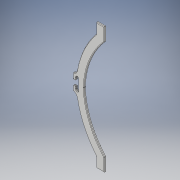
# Autodesk Inventor part: Baseplate_aussen_unten
Saved by Autodesk Inventor 2018 (Build 220112000, 112)
## iProperties
Created: 2020-01-15
Part Number: Baseplate_aussen_unten
Material: Generisch
Document SubType Name: Modeling
Designer: maxse
Density: 1 g/cm^3
Appearance: Vorgabe
Author: maxse
Autodesk Inventor part; units mm, degrees
ref_plane "YZ Plane" through (0, 0, 0) normal (1, 0, 0) x (0, 1, 0)
ref_plane "XZ Plane" through (0, 0, 0) normal (0, 1, 0) x (-1, 0, 0)
ref_plane "XY Plane" through (0, 0, 0) normal (0, 0, 1) x (1, 0, 0)
sketch "Skizze1" plane through (0, 0, 0) normal (0, 1, 0) x (-1, 0, 0)
  arc A0 (39, 0) -> (0, 95) centre (-110.879, -6.024) ccw
  line L0 (0, 95) -> (0, 120)
  line L1 (0, 120) -> (15, 120)
  line L2 (15, 120) -> (15, 100.6336)
  arc A1 (54, 0) -> (15, 100.6336) centre (-110.879, -6.024) ccw
  line L3 (39, 0) -> (54, 0)
  line L4 (0, 0) -> (39, 0)
  line L5 (59, 0) -> (59, 15)
  line L6 (59, 15) -> (52.765, 15)
  line L7 (59, 0) -> (54, 0)
  dimension "d0" = 25
  dimension "d2" = 15
  dimension "d4" = 54
  dimension "d5" = 0
  dimension "d6" = 120
  dimension "d7" = 150
  dimension "d9" = 5
  dimension "d10" = 15
  dimension "d11" = 15
  constraints: 16 end point, 6 point on circle, 3 perpendicular, 2 centre point, 2 horizontal, 2 vertical, 1 collinear, 1 concentric
  measures "d0" distance of L0.start L0.end
  measures "d2" distance of L0.end L1.end
  measures "d4" distance of L3.end L4.start
  measures "d5" distance from line of L4.start L0
  measures "d6" distance from line of L4.start L1
  measures "d7" radius of A0
  measures "d9" distance of L3.end L5.start
  measures "d10" distance of L3.end L3.start
  measures "d11" distance of L5.start L5.end
extrude "Extrusion1" add sketch "Skizze1" along normal blind 4
mirror "Spiegeln1" about plane through (-54, 0, 0) normal (0, 0, -1) of "Extrusion1"
sketch "Skizze2" plane through (0, 0, 0) normal (0, -1, 0) x (1, 0, 0)
  line L0 (-59, 15) -> (-59, -15) projected
  line L1 (-59, -5) -> (-54, -5)
  line L2 (-54, -5) -> (-54, -9.5)
  line L3 (-59, 5) -> (-54, 5)
  line L4 (-54, 5) -> (-54, 9.5)
  line L5 (-49, -9.5) -> (-49, 9.5)
  arc A0 (-49, 9.5) -> (-54, 9.5) centre (-51.5, 9.5) ccw
  arc A1 (-54, -9.5) -> (-49, -9.5) centre (-51.5, -9.5) ccw
  point P0 (0, 0)
  dimension "d15" = 10
  dimension "d16" = 5
  dimension "d17" = 10
  dimension "d18" = 5
  dimension "d19" = 5
  dimension "d20" = 24
  dimension "d21" = 4.5
  constraints: 10 end point, 4 point on circle, 4 tangent, 2 centre point, 2 horizontal, 2 point on line, 2 vertical, 1 perpendicular
  measures "d15" distance between parallel lines of L5 L0
  measures "d16" distance between parallel lines of L5 L2
  measures "d17" distance between parallel lines of L3 L1
  measures "d18" distance of L3.start L3.end
  measures "d19" distance from line of point (0, 0) L3
  measures "d21" distance from line of L1 A1.centre
extrude "Extrusion2" cut sketch "Skizze2" against normal blind 4
fillet "Rundung1" radius 10 3 edges at (-52.765, 2, -15) (-52.765, 2, 15) (-39, 2, 0)
fillet "Rundung2" radius 1 46 edges at (-7.5, 4, -120) (0, 4, -107.5) (-15, 4, -110.3168) (-7.5, 0, -120) (0, 0, -107.5) (-15, 0, -110.3168) (-54.0935, 4, -17.8718) (-38.4134, 4, -64.2123) (-54.0935, 0, -17.8718) (-38.4134, 0, -64.2123) (-38.9913, 4, 0) (-27.8012, 4, 51.1406) (-27.8012, 4, -51.1406) (-38.9913, 0, 0) (-27.8012, 0, 51.1406) (-27.8012, 0, -51.1406) (-54.0935, 4, 17.8718) (-38.4134, 4, 64.2123) (-54.0935, 0, 17.8718) (-38.4134, 0, 64.2123) (-59, 4, 10) (-59, 0, 10) (-59, 0, -10) (-59, 4, -10) (-59, 2, -5) (-59, 2, 5) (-54, 2, 5) (-54, 2, -5) (-56.5, 4, -5) (-56.5, 4, 5) (-51.5, 4, 12) (-54, 4, 7.25) (-51.5, 4, -12) (-54, 4, -7.25) (-49, 4, 0) (-51.5, 0, -12) (-54, 0, -7.25) (-51.5, 0, 12) (-54, 0, 7.25) (-49, 0, 0) (-15, 4, 110.3168) (-15, 0, 110.3168) (-7.5, 4, 120) (-7.5, 0, 120) (0, 0, 107.5) (0, 4, 107.5)
sketch "Skizze3" plane through (0, 4, 0) normal (0, 1, 0) x (1, 0, 0)
  line L0 (-42.3353, -14.0715) -> (-42.3353, -14.5367)
  line L1 (-42.3353, -14.5367) -> (-45.3503, -14.5367)
  line L2 (-45.3503, -14.5367) -> (-43.2996, -15.45)
  line L3 (-43.2996, -15.45) -> (-43.2996, -15.7336)
  line L4 (-43.2996, -15.7336) -> (-45.3503, -16.6384)
  line L5 (-45.3503, -16.6384) -> (-42.3353, -16.6384)
  line L6 (-42.3353, -16.6384) -> (-42.3353, -17.0724)
  line L7 (-42.3353, -17.0724) -> (-45.8353, -17.0724)
  line L8 (-45.8353, -17.0724) -> (-45.8353, -16.437)
  line L9 (-45.8353, -16.437) -> (-43.8867, -15.5634)
  line L10 (-43.8867, -15.5634) -> (-45.8353, -14.7182)
  line L11 (-45.8353, -14.7182) -> (-45.8353, -14.0715)
  line L12 (-45.8353, -14.0715) -> (-42.3353, -14.0715)
  spline S0 degree 2 poles (-42.6132, -11.933) (-42.5735, -11.9869) (-42.4317, -12.1684) (-42.3892, -12.2535) knots 0 0 0 1 2 2 2
  spline S1 degree 2 poles (-42.3892, -12.2535) (-42.3268, -12.3698) (-42.2615, -12.5882) (-42.2615, -12.7867) knots 0 0 0 1 2 2 2
  spline S2 degree 2 poles (-42.2615, -12.7867) (-42.2615, -12.9484) (-42.3835, -13.2405) (-42.4941, -13.3511) knots 0 0 0 1 2 2 2
  spline S3 degree 2 poles (-42.4941, -13.3511) (-42.6019, -13.4561) (-42.9196, -13.5837) (-43.0954, -13.5837) knots 0 0 0 1 2 2 2
  spline S4 degree 2 poles (-43.0954, -13.5837) (-43.3677, -13.5837) (-43.7534, -13.354) (-43.8641, -13.1044) knots 0 0 0 1 2 2 2
  spline S5 degree 2 poles (-43.8641, -13.1044) (-43.9662, -12.8831) (-44.0427, -12.2818) (-44.0626, -11.933) knots 0 0 0 1 2 2 2
  line L13 (-44.0626, -11.933) -> (-44.1477, -11.933)
  spline S6 degree 2 poles (-44.1477, -11.933) (-44.3008, -11.933) (-44.4909, -12.0266) (-44.5448, -12.1117) knots 0 0 0 1 2 2 2
  spline S7 degree 2 poles (-44.5448, -12.1117) (-44.5987, -12.1968) (-44.6327, -12.4407) (-44.6327, -12.5711) knots 0 0 0 1 2 2 2
  spline S8 degree 2 poles (-44.6327, -12.5711) (-44.6327, -12.7243) (-44.5419, -13.1384) (-44.454, -13.3455) knots 0 0 0 1 2 2 2
  line L14 (-44.454, -13.3455) -> (-44.454, -13.371)
  line L15 (-44.454, -13.371) -> (-44.905, -13.371)
  spline S9 degree 2 poles (-44.905, -13.371) (-44.939, -13.249) (-45.0241, -12.7924) (-45.0241, -12.5683) knots 0 0 0 1 2 2 2
  spline S10 degree 2 poles (-45.0241, -12.5683) (-45.0241, -12.296) (-44.939, -11.9245) (-44.8284, -11.777) knots 0 0 0 1 2 2 2
  spline S11 degree 2 poles (-44.8284, -11.777) (-44.7206, -11.6323) (-44.3774, -11.4905) (-44.1307, -11.4905) knots 0 0 0 1 2 2 2
  line L16 (-44.1307, -11.4905) -> (-42.3353, -11.4905)
  line L17 (-42.3353, -11.4905) -> (-42.3353, -11.933)
  line L18 (-42.3353, -11.933) -> (-42.6132, -11.933)
  line L19 (-42.982, -11.933) -> (-43.7109, -11.933)
  spline S12 degree 2 poles (-43.7109, -11.933) (-43.6967, -12.0918) (-43.6485, -12.5711) (-43.6031, -12.7215) knots 0 0 0 1 2 2 2
  spline S13 degree 2 poles (-43.6031, -12.7215) (-43.5492, -12.8973) (-43.3252, -13.1271) (-43.1266, -13.1271) knots 0 0 0 1 2 2 2
  spline S14 degree 2 poles (-43.1266, -13.1271) (-42.8997, -13.1271) (-42.67, -12.8718) (-42.67, -12.6279) knots 0 0 0 1 2 2 2
  spline S15 degree 2 poles (-42.67, -12.6279) (-42.67, -12.4208) (-42.8487, -12.0805) (-42.982, -11.933) knots 0 0 0 1 2 2 2
  line L20 (-42.3353, -8.8301) -> (-42.3353, -9.3718)
  line L21 (-42.3353, -9.3718) -> (-43.3223, -10.01)
  line L22 (-43.3223, -10.01) -> (-42.3353, -10.6651)
  line L23 (-42.3353, -10.6651) -> (-42.3353, -11.1672)
  line L24 (-42.3353, -11.1672) -> (-43.6372, -10.2567)
  line L25 (-43.6372, -10.2567) -> (-44.9617, -11.1587)
  line L26 (-44.9617, -11.1587) -> (-44.9617, -10.6169)
  line L27 (-44.9617, -10.6169) -> (-43.9832, -9.9816)
  line L28 (-43.9832, -9.9816) -> (-44.9617, -9.3321)
  line L29 (-44.9617, -9.3321) -> (-44.9617, -8.8301)
  line L30 (-44.9617, -8.8301) -> (-43.6655, -9.7348)
  line L31 (-43.6655, -9.7348) -> (-42.3353, -8.8301)
  spline S16 degree 2 poles (-42.2729, -5.9739) (-42.2729, -6.354) (-42.4317, -6.8872) (-42.5452, -7.1226) knots 0 0 0 1 2 2 2
  line L32 (-42.5452, -7.1226) -> (-43.1295, -7.1226)
  line L33 (-43.1295, -7.1226) -> (-43.1295, -7.0886)
  spline S17 degree 2 poles (-43.1295, -7.0886) (-42.9139, -6.8588) (-42.6756, -6.2774) (-42.6756, -6.0079) knots 0 0 0 1 2 2 2
  spline S18 degree 2 poles (-42.6756, -6.0079) (-42.6756, -5.6222) (-42.9961, -5.2279) (-43.2599, -5.2279) knots 0 0 0 1 2 2 2
  spline S19 degree 2 poles (-43.2599, -5.2279) (-43.4698, -5.2279) (-43.7307, -5.435) (-43.796, -5.6591) knots 0 0 0 1 2 2 2
  spline S20 degree 2 poles (-43.796, -5.6591) (-43.8414, -5.8207) (-43.9038, -6.0902) (-43.9548, -6.2916) knots 0 0 0 1 2 2 2
  spline S21 degree 2 poles (-43.9548, -6.2916) (-44.003, -6.4731) (-44.1477, -6.7596) (-44.264, -6.8702) knots 0 0 0 1 2 2 2
  spline S22 degree 2 poles (-44.264, -6.8702) (-44.3803, -6.9779) (-44.6923, -7.0971) (-44.8965, -7.0971) knots 0 0 0 1 2 2 2
  spline S23 degree 2 poles (-44.8965, -7.0971) (-45.3219, -7.0971) (-45.8977, -6.4334) (-45.8977, -5.92) knots 0 0 0 1 2 2 2
  spline S24 degree 2 poles (-45.8977, -5.92) (-45.8977, -5.625) (-45.7814, -5.1032) (-45.6708, -4.8791) knots 0 0 0 1 2 2 2
  line L34 (-45.6708, -4.8791) -> (-45.1149, -4.8791)
  line L35 (-45.1149, -4.8791) -> (-45.1149, -4.9131)
  spline S25 degree 2 poles (-45.1149, -4.9131) (-45.268, -5.0805) (-45.4949, -5.6023) (-45.4949, -5.8888) knots 0 0 0 1 2 2 2
  spline S26 degree 2 poles (-45.4949, -5.8888) (-45.4949, -6.2121) (-45.1914, -6.6121) (-44.9447, -6.6121) knots 0 0 0 1 2 2 2
  spline S27 degree 2 poles (-44.9447, -6.6121) (-44.7235, -6.6121) (-44.4597, -6.3767) (-44.4001, -6.1554) knots 0 0 0 1 2 2 2
  spline S28 degree 2 poles (-44.4001, -6.1554) (-44.3604, -6.0079) (-44.2583, -5.5797) (-44.2158, -5.4378) knots 0 0 0 1 2 2 2
  spline S29 degree 2 poles (-44.2158, -5.4378) (-44.1051, -5.0776) (-43.6598, -4.7429) (-43.3337, -4.7429) knots 0 0 0 1 2 2 2
  spline S30 degree 2 poles (-43.3337, -4.7429) (-43.1266, -4.7429) (-42.7295, -4.9103) (-42.5906, -5.0606) knots 0 0 0 1 2 2 2
  spline S31 degree 2 poles (-42.5906, -5.0606) (-42.4374, -5.2279) (-42.2729, -5.6534) (-42.2729, -5.9739) knots 0 0 0 1 2 2 2
  spline S32 degree 2 poles (-42.2757, -3.1631) (-42.2757, -3.7928) (-42.982, -4.4848) (-43.6343, -4.4848) knots 0 0 0 1 2 2 2
  spline S33 degree 2 poles (-43.6343, -4.4848) (-44.2753, -4.4848) (-45.0354, -3.8126) (-45.0354, -3.2709) knots 0 0 0 1 2 2 2
  spline S34 degree 2 poles (-45.0354, -3.2709) (-45.0354, -3.027) (-44.8936, -2.6497) (-44.7433, -2.5108) knots 0 0 0 1 2 2 2
  spline S35 degree 2 poles (-44.7433, -2.5108) (-44.593, -2.369) (-44.159, -2.2186) (-43.8442, -2.2186) knots 0 0 0 1 2 2 2
  line L36 (-43.8442, -2.2186) -> (-43.6031, -2.2186)
  line L37 (-43.6031, -2.2186) -> (-43.6031, -4.0367)
  spline S36 degree 2 poles (-43.6031, -4.0367) (-43.1465, -4.0367) (-42.6615, -3.5772) (-42.6615, -3.1688) knots 0 0 0 1 2 2 2
  spline S37 degree 2 poles (-42.6615, -3.1688) (-42.6615, -3.0241) (-42.7267, -2.7433) (-42.7778, -2.6299) knots 0 0 0 1 2 2 2
  spline S38 degree 2 poles (-42.7778, -2.6299) (-42.8345, -2.5108) (-42.9337, -2.3463) (-42.9791, -2.2924) knots 0 0 0 1 2 2 2
  line L38 (-42.9791, -2.2924) -> (-42.9791, -2.2668)
  line L39 (-42.9791, -2.2668) -> (-42.497, -2.2668)
  spline S39 degree 2 poles (-42.497, -2.2668) (-42.4658, -2.3434) (-42.375, -2.576) (-42.3495, -2.6668) knots 0 0 0 1 2 2 2
  spline S40 degree 2 poles (-42.3495, -2.6668) (-42.3126, -2.7944) (-42.2757, -3.0043) (-42.2757, -3.1631) knots 0 0 0 1 2 2 2
  spline S41 degree 2 poles (-43.9406, -2.6497) (-44.1193, -2.6554) (-44.3803, -2.7292) (-44.4682, -2.8001) knots 0 0 0 1 2 2 2
  spline S42 degree 2 poles (-44.4682, -2.8001) (-44.5675, -2.8767) (-44.6724, -3.1177) (-44.6724, -3.2964) knots 0 0 0 1 2 2 2
  spline S43 degree 2 poles (-44.6724, -3.2964) (-44.6724, -3.4723) (-44.5675, -3.719) (-44.4654, -3.8211) knots 0 0 0 1 2 2 2
  spline S44 degree 2 poles (-44.4654, -3.8211) (-44.3604, -3.9204) (-44.108, -4.0225) (-43.9406, -4.0367) knots 0 0 0 1 2 2 2
  line L40 (-43.9406, -4.0367) -> (-43.9406, -2.6497)
  spline S45 degree 2 poles (-42.2729, -1.0614) (-42.2729, -1.3252) (-42.4147, -1.7818) (-42.4941, -1.9322) knots 0 0 0 1 2 2 2
  line L41 (-42.4941, -1.9322) -> (-42.9905, -1.9322)
  line L42 (-42.9905, -1.9322) -> (-42.9905, -1.9095)
  spline S46 degree 2 poles (-42.9905, -1.9095) (-42.9451, -1.8527) (-42.8373, -1.6996) (-42.7778, -1.572) knots 0 0 0 1 2 2 2
  spline S47 degree 2 poles (-42.7778, -1.572) (-42.7239, -1.4613) (-42.6444, -1.1891) (-42.6444, -1.0444) knots 0 0 0 1 2 2 2
  spline S48 degree 2 poles (-42.6444, -1.0444) (-42.6444, -0.9395) (-42.6927, -0.6984) (-42.7324, -0.6416) knots 0 0 0 1 2 2 2
  spline S49 degree 2 poles (-42.7324, -0.6416) (-42.7863, -0.5594) (-42.9082, -0.4856) (-43.033, -0.4856) knots 0 0 0 1 2 2 2
  spline S50 degree 2 poles (-43.033, -0.4856) (-43.189, -0.4856) (-43.3507, -0.6558) (-43.4046, -0.8742) knots 0 0 0 1 2 2 2
  spline S51 degree 2 poles (-43.4046, -0.8742) (-43.4244, -0.9593) (-43.4812, -1.2316) (-43.5124, -1.3479) knots 0 0 0 1 2 2 2
  spline S52 degree 2 poles (-43.5124, -1.3479) (-43.6003, -1.6485) (-43.9633, -1.9208) (-44.2214, -1.9208) knots 0 0 0 1 2 2 2
  spline S53 degree 2 poles (-44.2214, -1.9208) (-44.5788, -1.9208) (-45.0241, -1.3848) (-45.0241, -0.9423) knots 0 0 0 1 2 2 2
  spline S54 degree 2 poles (-45.0241, -0.9423) (-45.0241, -0.7239) (-44.9163, -0.2814) (-44.8341, -0.1311) knots 0 0 0 1 2 2 2
  line L43 (-44.8341, -0.1311) -> (-44.3604, -0.1311)
  line L44 (-44.3604, -0.1311) -> (-44.3604, -0.1538)
  spline S55 degree 2 poles (-44.3604, -0.1538) (-44.4966, -0.324) (-44.6525, -0.7381) (-44.6525, -0.9508) knots 0 0 0 1 2 2 2
  spline S56 degree 2 poles (-44.6525, -0.9508) (-44.6525, -1.1692) (-44.4682, -1.4698) (-44.2838, -1.4698) knots 0 0 0 1 2 2 2
  spline S57 degree 2 poles (-44.2838, -1.4698) (-44.1165, -1.4698) (-43.9548, -1.2912) (-43.9038, -1.0926) knots 0 0 0 1 2 2 2
  spline S58 degree 2 poles (-43.9038, -1.0926) (-43.8782, -0.9962) (-43.8272, -0.7523) (-43.796, -0.619) knots 0 0 0 1 2 2 2
  spline S59 degree 2 poles (-43.796, -0.619) (-43.7222, -0.3297) (-43.3847, -0.0347) (-43.0926, -0.0347) knots 0 0 0 1 2 2 2
  spline S60 degree 2 poles (-43.0926, -0.0347) (-42.9224, -0.0347) (-42.6218, -0.168) (-42.5111, -0.2985) knots 0 0 0 1 2 2 2
  spline S61 degree 2 poles (-42.5111, -0.2985) (-42.3948, -0.4374) (-42.2729, -0.792) (-42.2729, -1.0614) knots 0 0 0 1 2 2 2
  spline S62 degree 2 poles (-42.2729, 1.0857) (-42.2729, 0.8219) (-42.4147, 0.3652) (-42.4941, 0.2149) knots 0 0 0 1 2 2 2
  line L45 (-42.4941, 0.2149) -> (-42.9905, 0.2149)
  line L46 (-42.9905, 0.2149) -> (-42.9905, 0.2376)
  spline S63 degree 2 poles (-42.9905, 0.2376) (-42.9451, 0.2943) (-42.8373, 0.4475) (-42.7778, 0.5751) knots 0 0 0 1 2 2 2
  spline S64 degree 2 poles (-42.7778, 0.5751) (-42.7239, 0.6857) (-42.6444, 0.958) (-42.6444, 1.1027) knots 0 0 0 1 2 2 2
  spline S65 degree 2 poles (-42.6444, 1.1027) (-42.6444, 1.2076) (-42.6927, 1.4487) (-42.7324, 1.5054) knots 0 0 0 1 2 2 2
  spline S66 degree 2 poles (-42.7324, 1.5054) (-42.7863, 1.5877) (-42.9082, 1.6614) (-43.033, 1.6614) knots 0 0 0 1 2 2 2
  spline S67 degree 2 poles (-43.033, 1.6614) (-43.189, 1.6614) (-43.3507, 1.4913) (-43.4046, 1.2729) knots 0 0 0 1 2 2 2
  spline S68 degree 2 poles (-43.4046, 1.2729) (-43.4244, 1.1878) (-43.4812, 0.9155) (-43.5124, 0.7992) knots 0 0 0 1 2 2 2
  spline S69 degree 2 poles (-43.5124, 0.7992) (-43.6003, 0.4985) (-43.9633, 0.2263) (-44.2214, 0.2263) knots 0 0 0 1 2 2 2
  spline S70 degree 2 poles (-44.2214, 0.2263) (-44.5788, 0.2263) (-45.0241, 0.7623) (-45.0241, 1.2048) knots 0 0 0 1 2 2 2
  spline S71 degree 2 poles (-45.0241, 1.2048) (-45.0241, 1.4232) (-44.9163, 1.8656) (-44.8341, 2.016) knots 0 0 0 1 2 2 2
  line L47 (-44.8341, 2.016) -> (-44.3604, 2.016)
  line L48 (-44.3604, 2.016) -> (-44.3604, 1.9933)
  spline S72 degree 2 poles (-44.3604, 1.9933) (-44.4966, 1.8231) (-44.6525, 1.409) (-44.6525, 1.1963) knots 0 0 0 1 2 2 2
  spline S73 degree 2 poles (-44.6525, 1.1963) (-44.6525, 0.9779) (-44.4682, 0.6772) (-44.2838, 0.6772) knots 0 0 0 1 2 2 2
  spline S74 degree 2 poles (-44.2838, 0.6772) (-44.1165, 0.6772) (-43.9548, 0.8559) (-43.9038, 1.0545) knots 0 0 0 1 2 2 2
  spline S75 degree 2 poles (-43.9038, 1.0545) (-43.8782, 1.1509) (-43.8272, 1.3948) (-43.796, 1.5281) knots 0 0 0 1 2 2 2
  spline S76 degree 2 poles (-43.796, 1.5281) (-43.7222, 1.8174) (-43.3847, 2.1124) (-43.0926, 2.1124) knots 0 0 0 1 2 2 2
  spline S77 degree 2 poles (-43.0926, 2.1124) (-42.9224, 2.1124) (-42.6218, 1.9791) (-42.5111, 1.8486) knots 0 0 0 1 2 2 2
  spline S78 degree 2 poles (-42.5111, 1.8486) (-42.3948, 1.7097) (-42.2729, 1.3551) (-42.2729, 1.0857) knots 0 0 0 1 2 2 2
  spline S79 degree 2 poles (-42.2757, 3.6639) (-42.2757, 3.0342) (-42.982, 2.3421) (-43.6343, 2.3421) knots 0 0 0 1 2 2 2
  spline S80 degree 2 poles (-43.6343, 2.3421) (-44.2753, 2.3421) (-45.0354, 3.0144) (-45.0354, 3.5561) knots 0 0 0 1 2 2 2
  spline S81 degree 2 poles (-45.0354, 3.5561) (-45.0354, 3.8) (-44.8936, 4.1772) (-44.7433, 4.3162) knots 0 0 0 1 2 2 2
  spline S82 degree 2 poles (-44.7433, 4.3162) (-44.593, 4.458) (-44.159, 4.6084) (-43.8442, 4.6084) knots 0 0 0 1 2 2 2
  line L49 (-43.8442, 4.6084) -> (-43.6031, 4.6084)
  line L50 (-43.6031, 4.6084) -> (-43.6031, 2.7903)
  spline S83 degree 2 poles (-43.6031, 2.7903) (-43.1465, 2.7903) (-42.6615, 3.2498) (-42.6615, 3.6582) knots 0 0 0 1 2 2 2
  spline S84 degree 2 poles (-42.6615, 3.6582) (-42.6615, 3.8028) (-42.7267, 4.0836) (-42.7778, 4.1971) knots 0 0 0 1 2 2 2
  spline S85 degree 2 poles (-42.7778, 4.1971) (-42.8345, 4.3162) (-42.9337, 4.4807) (-42.9791, 4.5346) knots 0 0 0 1 2 2 2
  line L51 (-42.9791, 4.5346) -> (-42.9791, 4.5601)
  line L52 (-42.9791, 4.5601) -> (-42.497, 4.5601)
  spline S86 degree 2 poles (-42.497, 4.5601) (-42.4658, 4.4836) (-42.375, 4.251) (-42.3495, 4.1602) knots 0 0 0 1 2 2 2
  spline S87 degree 2 poles (-42.3495, 4.1602) (-42.3126, 4.0326) (-42.2757, 3.8227) (-42.2757, 3.6639) knots 0 0 0 1 2 2 2
  spline S88 degree 2 poles (-43.9406, 4.1772) (-44.1193, 4.1716) (-44.3803, 4.0978) (-44.4682, 4.0269) knots 0 0 0 1 2 2 2
  spline S89 degree 2 poles (-44.4682, 4.0269) (-44.5675, 3.9503) (-44.6724, 3.7092) (-44.6724, 3.5306) knots 0 0 0 1 2 2 2
  spline S90 degree 2 poles (-44.6724, 3.5306) (-44.6724, 3.3547) (-44.5675, 3.1079) (-44.4654, 3.0058) knots 0 0 0 1 2 2 2
  spline S91 degree 2 poles (-44.4654, 3.0058) (-44.3604, 2.9066) (-44.108, 2.8045) (-43.9406, 2.7903) knots 0 0 0 1 2 2 2
  line L53 (-43.9406, 2.7903) -> (-43.9406, 4.1772)
  line L54 (-42.3353, 5.5075) -> (-42.3353, 5.065)
  line L55 (-42.3353, 5.065) -> (-45.9913, 5.065)
  line L56 (-45.9913, 5.065) -> (-45.9913, 5.5075)
  line L57 (-45.9913, 5.5075) -> (-42.3353, 5.5075)
  line L58 (-42.3353, 9.1351) -> (-43.8555, 9.1351)
  spline S92 degree 2 poles (-43.8555, 9.1351) (-44.0371, 9.1351) (-44.3462, 9.1067) (-44.4313, 9.0614) knots 0 0 0 1 2 2 2
  spline S93 degree 2 poles (-44.4313, 9.0614) (-44.5249, 9.016) (-44.6157, 8.843) (-44.6157, 8.6926) knots 0 0 0 1 2 2 2
  spline S94 degree 2 poles (-44.6157, 8.6926) (-44.6157, 8.5565) (-44.4483, 8.2445) (-44.2895, 8.08) knots 0 0 0 1 2 2 2
  spline S95 degree 2 poles (-44.2895, 8.08) (-44.2498, 8.0828) (-44.1392, 8.0885) (-44.0654, 8.0885) knots 0 0 0 1 2 2 2
  line L59 (-44.0654, 8.0885) -> (-42.3353, 8.0885)
  line L60 (-42.3353, 8.0885) -> (-42.3353, 7.646)
  line L61 (-42.3353, 7.646) -> (-43.8555, 7.646)
  spline S96 degree 2 poles (-43.8555, 7.646) (-44.0371, 7.646) (-44.3462, 7.6177) (-44.4313, 7.5723) knots 0 0 0 1 2 2 2
  spline S97 degree 2 poles (-44.4313, 7.5723) (-44.5249, 7.5269) (-44.6157, 7.3539) (-44.6157, 7.2036) knots 0 0 0 1 2 2 2
  spline S98 degree 2 poles (-44.6157, 7.2036) (-44.6157, 7.0618) (-44.437, 6.7469) (-44.298, 6.5994) knots 0 0 0 1 2 2 2
  line L62 (-44.298, 6.5994) -> (-42.3353, 6.5994)
  line L63 (-42.3353, 6.5994) -> (-42.3353, 6.157)
  line L64 (-42.3353, 6.157) -> (-44.9617, 6.157)
  line L65 (-44.9617, 6.157) -> (-44.9617, 6.5994)
  line L66 (-44.9617, 6.5994) -> (-44.6724, 6.5994)
  spline S99 degree 2 poles (-44.6724, 6.5994) (-44.8454, 6.7725) (-45.0354, 7.1128) (-45.0354, 7.317) knots 0 0 0 1 2 2 2
  spline S100 degree 2 poles (-45.0354, 7.317) (-45.0354, 7.5496) (-44.8227, 7.9098) (-44.5816, 8.0034) knots 0 0 0 1 2 2 2
  spline S101 degree 2 poles (-44.5816, 8.0034) (-44.8057, 8.2048) (-45.0354, 8.5849) (-45.0354, 8.8061) knots 0 0 0 1 2 2 2
  spline S102 degree 2 poles (-45.0354, 8.8061) (-45.0354, 8.9763) (-44.9305, 9.2542) (-44.8114, 9.3563) knots 0 0 0 1 2 2 2
  spline S103 degree 2 poles (-44.8114, 9.3563) (-44.6923, 9.4613) (-44.3349, 9.5776) (-44.0654, 9.5776) knots 0 0 0 1 2 2 2
  line L67 (-44.0654, 9.5776) -> (-42.3353, 9.5776)
  line L68 (-42.3353, 9.5776) -> (-42.3353, 9.1351)
  spline S104 degree 2 poles (-42.6132, 11.6622) (-42.5735, 11.6084) (-42.4317, 11.4268) (-42.3892, 11.3417) knots 0 0 0 1 2 2 2
  spline S105 degree 2 poles (-42.3892, 11.3417) (-42.3268, 11.2255) (-42.2615, 11.0071) (-42.2615, 10.8085) knots 0 0 0 1 2 2 2
  spline S106 degree 2 poles (-42.2615, 10.8085) (-42.2615, 10.6468) (-42.3835, 10.3547) (-42.4941, 10.2441) knots 0 0 0 1 2 2 2
  spline S107 degree 2 poles (-42.4941, 10.2441) (-42.6019, 10.1391) (-42.9196, 10.0115) (-43.0954, 10.0115) knots 0 0 0 1 2 2 2
  spline S108 degree 2 poles (-43.0954, 10.0115) (-43.3677, 10.0115) (-43.7534, 10.2413) (-43.8641, 10.4909) knots 0 0 0 1 2 2 2
  spline S109 degree 2 poles (-43.8641, 10.4909) (-43.9662, 10.7121) (-44.0427, 11.3134) (-44.0626, 11.6622) knots 0 0 0 1 2 2 2
  line L69 (-44.0626, 11.6622) -> (-44.1477, 11.6622)
  spline S110 degree 2 poles (-44.1477, 11.6622) (-44.3008, 11.6622) (-44.4909, 11.5686) (-44.5448, 11.4836) knots 0 0 0 1 2 2 2
  spline S111 degree 2 poles (-44.5448, 11.4836) (-44.5987, 11.3985) (-44.6327, 11.1545) (-44.6327, 11.0241) knots 0 0 0 1 2 2 2
  spline S112 degree 2 poles (-44.6327, 11.0241) (-44.6327, 10.8709) (-44.5419, 10.4568) (-44.454, 10.2498) knots 0 0 0 1 2 2 2
  line L70 (-44.454, 10.2498) -> (-44.454, 10.2242)
  line L71 (-44.454, 10.2242) -> (-44.905, 10.2242)
  spline S113 degree 2 poles (-44.905, 10.2242) (-44.939, 10.3462) (-45.0241, 10.8028) (-45.0241, 11.0269) knots 0 0 0 1 2 2 2
  spline S114 degree 2 poles (-45.0241, 11.0269) (-45.0241, 11.2992) (-44.939, 11.6708) (-44.8284, 11.8182) knots 0 0 0 1 2 2 2
  spline S115 degree 2 poles (-44.8284, 11.8182) (-44.7206, 11.9629) (-44.3774, 12.1047) (-44.1307, 12.1047) knots 0 0 0 1 2 2 2
  line L72 (-44.1307, 12.1047) -> (-42.3353, 12.1047)
  line L73 (-42.3353, 12.1047) -> (-42.3353, 11.6622)
  line L74 (-42.3353, 11.6622) -> (-42.6132, 11.6622)
  line L75 (-42.982, 11.6622) -> (-43.7109, 11.6622)
  spline S116 degree 2 poles (-43.7109, 11.6622) (-43.6967, 11.5034) (-43.6485, 11.0241) (-43.6031, 10.8738) knots 0 0 0 1 2 2 2
  spline S117 degree 2 poles (-43.6031, 10.8738) (-43.5492, 10.6979) (-43.3252, 10.4682) (-43.1266, 10.4682) knots 0 0 0 1 2 2 2
  spline S118 degree 2 poles (-43.1266, 10.4682) (-42.8997, 10.4682) (-42.67, 10.7234) (-42.67, 10.9673) knots 0 0 0 1 2 2 2
  spline S119 degree 2 poles (-42.67, 10.9673) (-42.67, 11.1744) (-42.8487, 11.5148) (-42.982, 11.6622) knots 0 0 0 1 2 2 2
  line L76 (-42.3353, 14.7879) -> (-42.3353, 14.3454)
  line L77 (-42.3353, 14.3454) -> (-43.8329, 14.3454)
  spline S120 degree 2 poles (-43.8329, 14.3454) (-44.0144, 14.3454) (-44.3264, 14.3114) (-44.42, 14.2603) knots 0 0 0 1 2 2 2
  spline S121 degree 2 poles (-44.42, 14.2603) (-44.5192, 14.2064) (-44.6157, 14.0135) (-44.6157, 13.849) knots 0 0 0 1 2 2 2
  spline S122 degree 2 poles (-44.6157, 13.849) (-44.6157, 13.6845) (-44.4398, 13.3357) (-44.298, 13.1683) knots 0 0 0 1 2 2 2
  line L78 (-44.298, 13.1683) -> (-42.3353, 13.1683)
  line L79 (-42.3353, 13.1683) -> (-42.3353, 12.7259)
  line L80 (-42.3353, 12.7259) -> (-44.9617, 12.7259)
  line L81 (-44.9617, 12.7259) -> (-44.9617, 13.1683)
  line L82 (-44.9617, 13.1683) -> (-44.6696, 13.1683)
  spline S123 degree 2 poles (-44.6696, 13.1683) (-44.8483, 13.3669) (-45.0354, 13.7498) (-45.0354, 13.9653) knots 0 0 0 1 2 2 2
  spline S124 degree 2 poles (-45.0354, 13.9653) (-45.0354, 14.3511) (-44.5249, 14.7879) (-44.0399, 14.7879) knots 0 0 0 1 2 2 2
  line L83 (-44.0399, 14.7879) -> (-42.3353, 14.7879)
  line L84 (-42.3353, 17.471) -> (-42.3353, 17.0285)
  line L85 (-42.3353, 17.0285) -> (-43.8329, 17.0285)
  spline S125 degree 2 poles (-43.8329, 17.0285) (-44.0144, 17.0285) (-44.3264, 16.9945) (-44.42, 16.9434) knots 0 0 0 1 2 2 2
  spline S126 degree 2 poles (-44.42, 16.9434) (-44.5192, 16.8896) (-44.6157, 16.6967) (-44.6157, 16.5322) knots 0 0 0 1 2 2 2
  spline S127 degree 2 poles (-44.6157, 16.5322) (-44.6157, 16.3677) (-44.4398, 16.0188) (-44.298, 15.8515) knots 0 0 0 1 2 2 2
  line L86 (-44.298, 15.8515) -> (-42.3353, 15.8515)
  line L87 (-42.3353, 15.8515) -> (-42.3353, 15.409)
  line L88 (-42.3353, 15.409) -> (-44.9617, 15.409)
  line L89 (-44.9617, 15.409) -> (-44.9617, 15.8515)
  line L90 (-44.9617, 15.8515) -> (-44.6696, 15.8515)
  spline S128 degree 2 poles (-44.6696, 15.8515) (-44.8483, 16.05) (-45.0354, 16.4329) (-45.0354, 16.6485) knots 0 0 0 1 2 2 2
  spline S129 degree 2 poles (-45.0354, 16.6485) (-45.0354, 17.0342) (-44.5249, 17.471) (-44.0399, 17.471) knots 0 0 0 1 2 2 2
  line L91 (-44.0399, 17.471) -> (-42.3353, 17.471)
  point P0 (0, 0)
  point P1 (-45.9913, -17.4269)
  constraints: 1 other
extrude "Extrusion3" add sketch "Skizze3" along normal blind 1
